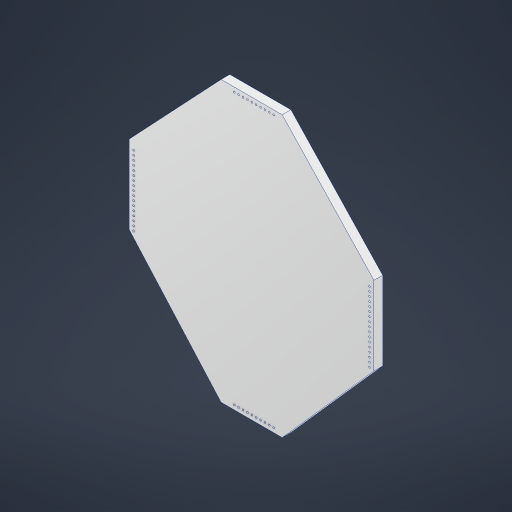
# Autodesk Inventor part: DVBS_008_bellypan
Saved by Autodesk Inventor 2024 (Build 280153000, 153)
## iProperties
Created: 2024-07-31
Part Number: DVBS_008_bellypan
Material: Aluminum 6061
Document SubType Name: Modeling
Designer: sarav
Density: 2.7 g/cm^3
Appearance: Aluminum - Flat
Author: sarav
Autodesk Inventor part; units mm, degrees
ref_plane "YZ Plane" through (0, 0, 0) normal (1, 0, 0) x (0, 1, 0)
ref_plane "XZ Plane" through (0, 0, 0) normal (0, 1, 0) x (-1, 0, 0)
ref_plane "XY Plane" through (0, 0, 0) normal (0, 0, 1) x (1, 0, 0)
sketch "Sketch1" plane through (0, 0, 0) normal (0, 0, 1) x (1, 0, 0)
  line L0 (0, 0) -> (0, 228.6)
  line L1 (711.2, 0) -> (711.2, 228.6)
  line L2 (266.7, -300.8863) -> (444.5, -300.8863)
  line L3 (355.6, 0) -> (355.6, 228.6)
  line L4 (266.7, 511.9137) -> (444.5, 511.9137)
  line L5 (266.7, 511.9137) -> (0, 228.6)
  line L6 (444.5, 511.9137) -> (711.2, 228.6)
  line L7 (711.2, 0) -> (444.5, -300.8863)
  line L8 (0, 0) -> (266.7, -300.8863)
  point P0 (355.6, -300.8863)
  point P1 (355.6, 511.9137)
  dimension "d39" = 228.6
  dimension "d40" = 711.2
  dimension "d41" = 177.8
  dimension "d42" = 355.6
  dimension "d43" = 177.8
  dimension "d46" = 812.8
  dimension "d47" = 300.8863
  constraints: 18 end point, 3 vertical, 2 horizontal, 2 midpoint, 2 point on line, 1 other
  measures "d39" distance of L0.start L0.end
  measures "d40" distance between parallel lines of L1 L0
  measures "d41" distance of L2.start L2.end
  measures "d42" distance between parallel lines of L3 L0
  measures "d43" distance of L4.start L4.end
  measures "d46" distance between parallel lines of L2 L4
  measures "d47" vertical distance of L1.start L2.end
extrude "Extrusion1" add sketch "Sketch1" along normal blind 25.4
sketch "Sketch3" plane through (0, 0, 25.4) normal (0, 0, 1) x (1, 0, 0)
  line L0 (444.5, -300.8863) -> (711.2, 0) projected
  line L1 (711.2, 0) -> (711.2, 228.6) projected
  line L2 (711.2, 228.6) -> (444.5, 511.9137) projected
  line L3 (444.5, 511.9137) -> (266.7, 511.9137) projected
  line L4 (266.7, 511.9137) -> (0, 228.6) projected
  line L5 (0, 228.6) -> (0, 0) projected
  line L6 (0, 0) -> (266.7, -300.8863) projected
  line L7 (266.7, -300.8863) -> (444.5, -300.8863) projected
  circle A0 centre (419.6269, 499.2137) radius 2.5019
  line L8 (254.7447, 499.2137) -> (456.4553, 499.2137) construction
  circle A1 centre (406.9269, 499.2137) radius 2.5019
  line L9 (242.0447, 499.2137) -> (443.7553, 499.2137) construction
  circle A2 centre (394.2269, 499.2137) radius 2.5019
  line L10 (229.3447, 499.2137) -> (431.0553, 499.2137) construction
  circle A3 centre (381.5269, 499.2137) radius 2.5019
  line L11 (216.6447, 499.2137) -> (418.3553, 499.2137) construction
  circle A4 centre (368.8269, 499.2137) radius 2.5019
  line L12 (203.9447, 499.2137) -> (405.6553, 499.2137) construction
  circle A5 centre (356.1269, 499.2137) radius 2.5019
  line L13 (191.2447, 499.2137) -> (392.9553, 499.2137) construction
  circle A6 centre (343.4269, 499.2137) radius 2.5019
  line L14 (178.5447, 499.2137) -> (380.2553, 499.2137) construction
  circle A7 centre (330.7269, 499.2137) radius 2.5019
  line L15 (165.8447, 499.2137) -> (367.5553, 499.2137) construction
  circle A8 centre (318.0269, 499.2137) radius 2.5019
  line L16 (153.1447, 499.2137) -> (354.8553, 499.2137) construction
  circle A9 centre (305.3269, 499.2137) radius 2.5019
  line L17 (140.4447, 499.2137) -> (342.1553, 499.2137) construction
  circle A10 centre (305.3269, -288.1863) radius 2.5019
  line L18 (305.3269, 499.2137) -> (305.3269, -288.1863) construction
  line L19 (257.0535, -288.1863) -> (455.757, -288.1863) construction
  circle A11 centre (318.0269, -288.1863) radius 2.5019
  line L20 (269.7535, -288.1863) -> (468.457, -288.1863) construction
  circle A12 centre (330.7269, -288.1863) radius 2.5019
  line L21 (282.4535, -288.1863) -> (481.157, -288.1863) construction
  circle A13 centre (343.4269, -288.1863) radius 2.5019
  line L22 (295.1535, -288.1863) -> (493.857, -288.1863) construction
  circle A14 centre (356.1269, -288.1863) radius 2.5019
  line L23 (307.8535, -288.1863) -> (506.557, -288.1863) construction
  circle A15 centre (368.8269, -288.1863) radius 2.5019
  line L24 (320.5535, -288.1863) -> (519.257, -288.1863) construction
  circle A16 centre (381.5269, -288.1863) radius 2.5019
  line L25 (333.2535, -288.1863) -> (531.957, -288.1863) construction
  circle A17 centre (394.2269, -288.1863) radius 2.5019
  line L26 (345.9535, -288.1863) -> (544.657, -288.1863) construction
  circle A18 centre (406.9269, -288.1863) radius 2.5019
  line L27 (358.6535, -288.1863) -> (557.357, -288.1863) construction
  circle A19 centre (419.6269, -288.1863) radius 2.5019
  line L28 (371.3535, -288.1863) -> (570.057, -288.1863) construction
  circle A20 centre (12.7, 206.4884) radius 2.5019
  line L29 (12.7, 242.0911) -> (12.7, -14.3279) construction
  circle A21 centre (12.7, 193.7884) radius 2.5019
  line L30 (12.7, 229.3911) -> (12.7, -27.0279) construction
  circle A22 centre (12.7, 181.0884) radius 2.5019
  line L31 (12.7, 216.6911) -> (12.7, -39.7279) construction
  circle A23 centre (12.7, 168.3884) radius 2.5019
  line L32 (12.7, 203.9911) -> (12.7, -52.4279) construction
  circle A24 centre (12.7, 155.6884) radius 2.5019
  line L33 (12.7, 191.2911) -> (12.7, -65.1279) construction
  circle A25 centre (12.7, 142.9884) radius 2.5019
  line L34 (12.7, 178.5911) -> (12.7, -77.8279) construction
  circle A26 centre (12.7, 130.2884) radius 2.5019
  line L35 (12.7, 165.8911) -> (12.7, -90.5279) construction
  circle A27 centre (12.7, 117.5884) radius 2.5019
  line L36 (12.7, 153.1911) -> (12.7, -103.2279) construction
  circle A28 centre (12.7, 104.8884) radius 2.5019
  line L37 (12.7, 140.4911) -> (12.7, -115.9279) construction
  circle A29 centre (12.7, 92.1884) radius 2.5019
  line L38 (12.7, 127.7911) -> (12.7, -128.6279) construction
  circle A30 centre (12.7, 79.4884) radius 2.5019
  line L39 (12.7, 115.0911) -> (12.7, -141.3279) construction
  circle A31 centre (12.7, 66.7884) radius 2.5019
  line L40 (12.7, 102.3911) -> (12.7, -154.0279) construction
  circle A32 centre (12.7, 54.0884) radius 2.5019
  line L41 (12.7, 89.6911) -> (12.7, -166.7279) construction
  circle A33 centre (12.7, 41.3884) radius 2.5019
  line L42 (12.7, 76.9911) -> (12.7, -179.4279) construction
  circle A34 centre (12.7, 28.6884) radius 2.5019
  line L43 (12.7, 64.2911) -> (12.7, -192.1279) construction
  circle A35 centre (12.7, 15.9884) radius 2.5019
  line L44 (12.7, 51.5911) -> (12.7, -204.8279) construction
  circle A36 centre (12.7, 3.2884) radius 2.5019
  line L45 (12.7, 38.8911) -> (12.7, -217.5279) construction
  circle A37 centre (12.7, -9.4116) radius 2.5019 construction
  line L46 (12.7, 26.1911) -> (12.7, -230.2279) construction
  circle A38 centre (698.5, 206.4884) radius 2.5019
  line L47 (12.7, 206.4884) -> (698.5, 206.4884) construction
  line L48 (698.5, 242.0911) -> (698.5, -14.3279) construction
  circle A39 centre (698.5, 193.7884) radius 2.5019
  circle A40 centre (698.5, 181.0884) radius 2.5019
  circle A41 centre (698.5, 168.3884) radius 2.5019
  circle A42 centre (698.5, 155.6884) radius 2.5019
  circle A43 centre (698.5, 142.9884) radius 2.5019
  circle A44 centre (698.5, 130.2884) radius 2.5019
  circle A45 centre (698.5, 117.5884) radius 2.5019
  circle A46 centre (698.5, 104.8884) radius 2.5019
  circle A47 centre (698.5, 92.1884) radius 2.5019
  circle A48 centre (698.5, 79.4884) radius 2.5019
  circle A49 centre (698.5, 66.7884) radius 2.5019
  circle A50 centre (698.5, 54.0884) radius 2.5019
  circle A51 centre (698.5, 41.3884) radius 2.5019
  circle A52 centre (698.5, 28.6884) radius 2.5019
  circle A53 centre (698.5, 15.9884) radius 2.5019
  circle A54 centre (698.5, 3.2884) radius 2.5019
  circle A55 centre (698.5, -9.4116) radius 2.5019 construction
  dimension "d48" = 5.0038
  dimension "d50" = 12.7
  dimension "d55" = 12.7
  dimension "d60" = 5.0038
  dimension "d61" = 12.7
  dimension "d64" = 12.7
  dimension "d69" = 5.0038
  dimension "d70" = 12.7
  dimension "d73" = 12.7
  dimension "d78" = 5.0038
  dimension "d79" = 12.7
  dimension "d82" = 12.7
  constraints: 82 end point, 56 centre point, 34 point on line, 6 horizontal, 5 vertical, 3 collinear, 1 parallel, 206 other
  measures "d48" diameter of A0
  measures "d50" distance from line of L3 A0.centre
  measures "d55" distance of A0.centre A1.centre
  measures "d60" diameter of A10
  measures "d61" distance from line of L7 L18.end
  measures "d64" distance of L18.end A11.centre
  measures "d69" diameter of A20
  measures "d70" distance from line of L5 L47.start
  measures "d73" distance of L47.start A21.centre
  measures "d78" diameter of A38
  measures "d79" distance from line of L1 L47.end
  measures "d82" distance of L47.end A39.centre
extrude "Extrusion2" cut sketch "Sketch3" against normal through all contours A0 | A1 | A2 | A3 | A4 | A5 | A6 | A7 | A8 | A9 | A10 | A11 | A12 | A13 | A14 | A15 | A16 | A17 | A18 | A19 | A20 | A21 | A22 | A23 | A24 | A25 | A26 | A27 | A28 | A29 | A30 | A31 | A32 | A33 | A34 | A35 | A36 | A38 | A39 | A40 | A41 | A42 | A43 | A44 | A45 | A46 | A47 | A48 | A49 | A50 | A51 | A52 | A53 | A54
body "Solid1"
